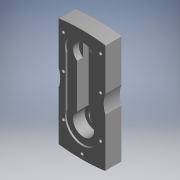
# Autodesk Inventor part: 1464690 EAMM-U-145-D100-...-348S---(OT)
Saved by Autodesk Inventor 2017.3 (Build 213256000, 256)
## iProperties
Part Number: 1464690 EAMM-U-145-D100-...-348S---(OT)
Material: Generic
Catalog Web Link: www.cadenas.de
Description: EAMM-U---(OT)-Fousing top part
Vendor: FESTO
Document SubType Name: Modeling
Designer: partserver
Manufacturer: FESTO
Mass: 1891.08 g
Surface Area: 1864.55 cm^2
Volume: 1891.08 cm^3
Density: 1 g/cm^3
Appearance: PSOLRGB-192-192-192
Category: PARTsolutions
Company: FESTO
Title: 1464690 EAMM-U-145-D100-...-348S---(OT)
Author: Cadenas PARTsolutions
Comments: Fousing top part
PSOL_IDENT_0: {$CADENAS_DATA\23d-libs\festo\parts\e\eamm\parts\eamm_u_ot.prj},226 {VTYP=3D},{NB=1464690 EAMM-U-145
PSOL_IDENT_1: -D100-...-348S---(OT)},{LINA=1464690 EAMM-U-145-D100-...-348S---(OT)},{NN=EAMM-U---(OT)},{DATE=27.10
PSOL_IDENT_2: .2020 09:44:40},{GEOMDATE=08.01.2020 14:15:00},{VERSION=},{LINEID=310},{WBVAR=},{WBNUMERIC=}  {NB=14
PSOL_IDENT_3: 64690 EAMM-U-145-D100-...-348S---(OT)},{LINA=1464690 EAMM-U-145-D100-...-348S---(OT)},{KT=DUMMY},{TN
PSOL_IDENT_4: R=1464690},{TYP=EAMM-U-145-D100-...-348S},{VERS=5S},{S=1},{B1=89.000},{D=-},{D1=0.000},{H0=188.000},
PSOL_IDENT_5: {H1=89.000},{H5=70.000},{H7=348.000},{H8=94.000},{H9=130.000},{H10=193.000},{T1=0.000},{T2=0.000}
NB: 1464690 EAMM-U-145-D100-...-348S---(OT)
NN: EAMM-U---(OT)
NT: Fousing top part
NBSYN: $TNR. $TYP.---(OT)
LINA: 1464690 EAMM-U-145-D100-...-348S---(OT)
CATALOG: Festo
TNR: 1464690
TYP: EAMM-U-145-D100-...-348S
VERS: 5S
B1: 89
D: -
D1: 0
H0: 188
H1: 89
H5: 70
H7: 348
H8: 94
H9: 130
H10: 193
T1: 0
T2: 0
SUPPLIER: FESTO
ARTICLENO: 1464690 EAMM-U-145-D100-...-348S---(OT)
BOMINFO: 1464690 EAMM-U-145-D100-...-348S---(OT)
CREATOR: CADENAS GmbH
Autodesk Inventor part; units mm, degrees
sketch "Sketch_1" plane through (0, 0, 0) normal (0, 1, 0) x (-1, 0, 0)
  line L0 (72.5, -155.8931) -> (72.5, -6.7735)
  arc A0 (72.5, -6.7735) -> (70.7696, -4.7917) centre (70.5, -6.7735) ccw
  arc A1 (70.7696, -4.7917) -> (-70.7696, -4.7917) centre (0, -525) ccw
  arc A2 (-70.7696, -4.7917) -> (-72.5, -6.7735) centre (-70.5, -6.7735) ccw
  line L1 (-72.5, -6.7735) -> (-72.5, -155.8931)
  arc A3 (-72.5, -155.8931) -> (-72.408, -156.4104) centre (-71, -155.8931) ccw
  arc A4 (-72.408, -211.5896) -> (-72.408, -156.4104) centre (-147.5, -184) ccw
  arc A5 (-72.408, -211.5896) -> (-72.5, -212.1069) centre (-71, -212.1069) ccw
  line L2 (-72.5, -212.1069) -> (-72.5, -341.2265)
  arc A6 (-72.5, -341.2265) -> (-70.7696, -343.2083) centre (-70.5, -341.2265) ccw
  arc A7 (-70.7696, -343.2083) -> (70.7696, -343.2083) centre (0, 177) ccw
  arc A8 (70.7696, -343.2083) -> (72.5, -341.2265) centre (70.5, -341.2265) ccw
  line L3 (72.5, -341.2265) -> (72.5, -212.1069)
  arc A9 (72.5, -212.1069) -> (72.408, -211.5896) centre (71, -212.1069) ccw
  arc A10 (72.408, -156.4104) -> (72.408, -211.5896) centre (147.5, -184) ccw
  arc A11 (72.408, -156.4104) -> (72.5, -155.8931) centre (71, -155.8931) ccw
  constraints: 24 point on circle, 12 centre point, 8 end point
extrude "Extrusion1" add sketch "Sketch_1" along normal blind 50
sketch "Sketch_12" plane through (0, 0, 0) normal (0, 1, 0) x (-1, 0, 0)
  arc A0 (20.3731, -115.3216) -> (-20.3731, -115.3216) centre (0, -90) ccw
  arc A1 (-20, -116.1008) -> (-20.3731, -115.3216) centre (-21, -116.1008) ccw
  line L0 (-20, -116.1008) -> (-20, -290.5)
  arc A2 (-20, -290.5) -> (20, -290.5) centre (0, -290.5) ccw
  line L1 (20, -290.5) -> (20, -116.1008)
  arc A3 (20.3731, -115.3216) -> (20, -116.1008) centre (21, -116.1008) ccw
  constraints: 8 point on circle, 4 centre point, 4 end point
extrude "Extrusion2" cut sketch "Sketch_12" along normal blind 41
sketch "Sketch_2" plane through (0, 0, 0) normal (0, 1, 0) x (-1, 0, 0)
  circle A0 centre (0, -278) radius 32.5
  constraints: 1 centre point
extrude "Extrusion3" cut sketch "Sketch_2" along normal blind 23
sketch "Sketch_3" plane through (0, 0, 0) normal (0, 1, 0) x (-1, 0, 0)
  circle A0 centre (0, -278) radius 20
  constraints: 1 centre point
extrude "Extrusion4" cut sketch "Sketch_3" along normal blind 45
sketch "Sketch_4" plane through (0, 0, 0) normal (0, 1, 0) x (-1, 0, 0)
  circle A0 centre (0, -90) radius 20
  constraints: 1 centre point
extrude "Extrusion5" cut sketch "Sketch_4" along normal blind 45
sketch "Sketch_21" plane through (0, 0, 0) normal (0, 1, 0) x (-1, 0, 0)
  arc A0 (50.0467, -105.8611) -> (-50.0467, -105.8611) centre (0, -90) ccw
  arc A1 (-50, -106.1632) -> (-50.0467, -105.8611) centre (-51, -106.1632) ccw
  line L0 (-50, -106.1632) -> (-50, -261.8368)
  arc A2 (-50.0467, -262.1389) -> (-50, -261.8368) centre (-51, -261.8368) ccw
  arc A3 (-50.0467, -262.1389) -> (50.0467, -262.1389) centre (0, -278) ccw
  arc A4 (50, -261.8368) -> (50.0467, -262.1389) centre (51, -261.8368) ccw
  line L1 (50, -261.8368) -> (50, -106.1632)
  arc A5 (50.0467, -105.8611) -> (50, -106.1632) centre (51, -106.1632) ccw
  constraints: 12 point on circle, 6 centre point, 4 end point
extrude "Extrusion6" cut sketch "Sketch_21" along normal blind 5
sketch "Sketch7" plane through (0, 50, 0) normal (0, 1, 0) x (1, 0, 0)
  point P0 (0, 15)
hole "Hole1" at (0, 50, -15) direction (0, -1, 0) diameter 9 depth 50 counterbore diameter 15 counterbore depth 9
sketch "Sketch8" plane through (0, 50, 0) normal (0, 1, 0) x (1, 0, 0)
  point P0 (57.5, 208)
hole "Hole2" at (57.5, 50, -208) direction (0, -1, 0) diameter 9 depth 50 counterbore diameter 15 counterbore depth 9
sketch "Sketch9" plane through (0, 50, 0) normal (0, 1, 0) x (1, 0, 0)
  point P0 (57.5, 313)
hole "Hole3" at (57.5, 50, -313) direction (0, -1, 0) diameter 9 depth 50 counterbore diameter 15 counterbore depth 9
sketch "Sketch10" plane through (0, 50, 0) normal (0, 1, 0) x (1, 0, 0)
  point P0 (57.5, 78)
hole "Hole4" at (57.5, 50, -78) direction (0, -1, 0) diameter 9 depth 50 counterbore diameter 15 counterbore depth 9
sketch "Sketch11" plane through (0, 50, 0) normal (0, 1, 0) x (1, 0, 0)
  point P0 (-57.5, 208)
hole "Hole5" at (-57.5, 50, -208) direction (0, -1, 0) diameter 9 depth 50 counterbore diameter 15 counterbore depth 9
sketch "Sketch12" plane through (0, 50, 0) normal (0, 1, 0) x (1, 0, 0)
  point P0 (-57.5, 313)
hole "Hole6" at (-57.5, 50, -313) direction (0, -1, 0) diameter 9 depth 50 counterbore diameter 15 counterbore depth 9
sketch "Sketch13" plane through (0, 50, 0) normal (0, 1, 0) x (1, 0, 0)
  point P0 (-57.5, 78)
hole "Hole7" at (-57.5, 50, -78) direction (0, -1, 0) diameter 9 depth 50 counterbore diameter 15 counterbore depth 9
sketch "Sketch14" plane through (0, 50, 0) normal (0, 1, 0) x (1, 0, 0)
  point P0 (44.5, 322.5)
hole "Hole8" at (44.5, 50, -322.5) direction (0, -1, 0) diameter 8.376 depth 30 tip angle 120 countersink diameter 10 countersink angle 90 thread size "M10x1.5" class "6H" standard "ISO Metric profile"
sketch "Sketch15" plane through (0, 50, 0) normal (0, 1, 0) x (1, 0, 0)
  point P0 (-44.5, 322.5)
hole "Hole9" at (-44.5, 50, -322.5) direction (0, -1, 0) diameter 8.376 depth 30 tip angle 120 countersink diameter 10 countersink angle 90 thread size "M10x1.5" class "6H" standard "ISO Metric profile"
sketch "Sketch16" plane through (0, 50, 0) normal (0, 1, 0) x (1, 0, 0)
  point P0 (44.5, 233.5)
hole "Hole10" at (44.5, 50, -233.5) direction (0, -1, 0) diameter 8.376 depth 30 tip angle 120 countersink diameter 10 countersink angle 90 thread size "M10x1.5" class "6H" standard "ISO Metric profile"
sketch "Sketch17" plane through (0, 50, 0) normal (0, 1, 0) x (1, 0, 0)
  point P0 (-44.5, 233.5)
hole "Hole11" at (-44.5, 50, -233.5) direction (0, -1, 0) diameter 8.376 depth 30 tip angle 120 countersink diameter 10 countersink angle 90 thread size "M10x1.5" class "6H" standard "ISO Metric profile"
ref_plane "ANBAU_XY" through (0, 0, -278) normal (0, 1, 0) x (1, 0, 0)
ref_plane "ANBAU_YZ" through (0, 0, -278) normal (1, 0, 0) x (0, 0, -1)
ref_plane "ANBAU_ZX" through (0, 0, -278) normal (0, 0, -1) x (0, 1, 0)
ref_plane "S1_1_XY" through (57.5, 41, -313) normal (0, 1, 0) x (1, 0, 0)
ref_plane "S1_1_YZ" through (57.5, 41, -313) normal (1, 0, 0) x (0, 0, -1)
ref_plane "S1_1_ZX" through (57.5, 41, -313) normal (0, 0, -1) x (0, 1, 0)
ref_plane "S1_2_XY" through (57.5, 41, -208) normal (0, 1, 0) x (1, 0, 0)
ref_plane "S1_2_YZ" through (57.5, 41, -208) normal (1, 0, 0) x (0, 0, -1)
ref_plane "S1_2_ZX" through (57.5, 41, -208) normal (0, 0, -1) x (0, 1, 0)
ref_plane "S1_3_XY" through (57.5, 41, -78) normal (0, 1, 0) x (1, 0, 0)
ref_plane "S1_3_YZ" through (57.5, 41, -78) normal (1, 0, 0) x (0, 0, -1)
ref_plane "S1_3_ZX" through (57.5, 41, -78) normal (0, 0, -1) x (0, 1, 0)
ref_plane "S2_1_XY" through (-57.5, 41, -313) normal (0, 1, 0) x (1, 0, 0)
ref_plane "S2_1_YZ" through (-57.5, 41, -313) normal (1, 0, 0) x (0, 0, -1)
ref_plane "S2_1_ZX" through (-57.5, 41, -313) normal (0, 0, -1) x (0, 1, 0)
ref_plane "S2_2_XY" through (-57.5, 41, -208) normal (0, 1, 0) x (1, 0, 0)
ref_plane "S2_2_YZ" through (-57.5, 41, -208) normal (1, 0, 0) x (0, 0, -1)
ref_plane "S2_2_ZX" through (-57.5, 41, -208) normal (0, 0, -1) x (0, 1, 0)
ref_plane "S2_3_XY" through (-57.5, 41, -78) normal (0, 1, 0) x (1, 0, 0)
ref_plane "S2_3_YZ" through (-57.5, 41, -78) normal (1, 0, 0) x (0, 0, -1)
ref_plane "S2_3_ZX" through (-57.5, 41, -78) normal (0, 0, -1) x (0, 1, 0)
ref_plane "S3_XY" through (0, 41, -15) normal (0, 1, 0) x (1, 0, 0)
ref_plane "S3_YZ" through (0, 41, -15) normal (1, 0, 0) x (0, 0, -1)
ref_plane "S3_ZX" through (0, 41, -15) normal (0, 0, -1) x (0, 1, 0)
body "Solid1"
